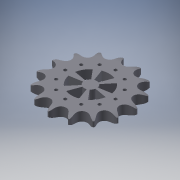
# Autodesk Inventor part: outer_drive_sprocket
Saved by Autodesk Inventor 2016 (Build 200138000, 138)
## iProperties
Created: 2016-11-04
Part Number: outer_drive_sprocket
Material: Steel
Document SubType Name: Modeling
Designer: hesaon
Density: 1 g/cm^3
Appearance: Steel
CustomPartVersion: 1
Author: hesaon
Autodesk Inventor part; units mm, degrees
ref_plane "YZ Plane" through (0, 0, 0) normal (1, 0, 0) x (0, 1, 0)
ref_plane "XZ Plane" through (0, 0, 0) normal (0, 1, 0) x (-1, 0, 0)
ref_plane "XY Plane" through (0, 0, 0) normal (0, 0, 1) x (1, 0, 0)
sketch "Theoretical Tooth Profile" plane through (0, 0, 0) normal (0, 0, 1) x (1, 0, 0)
  circle A0 centre (0, 0) radius 30.5418 construction
  line L0 (0, 0) -> (0, 30.5418) construction
  line L1 (0, 0) -> (12.4225, 27.9013) construction
  circle A1 centre (0, 0) radius 33.6844
  arc A2 (-3.3398, 27.8373) -> (3.3398, 27.8373) centre (0, 30.5418) ccw
  line L2 (0, 30.5418) -> (12.4225, 27.9013) construction
  line L3 (0, 30.5418) -> (5.2908, 34.8262) construction
  line L4 (5.2908, 34.8262) -> (-4.796, 30.1797) construction
  arc A3 (6.5675, 33.038) -> (5.1927, 31.041) centre (11.6537, 28.0648) ccw
  arc A4 (-5.1927, 31.041) -> (-6.5675, 33.038) centre (-11.6537, 28.0648) ccw
  line L5 (-11.6537, 28.0648) -> (-5.1927, 31.041) construction
  arc A5 (-4.796, 30.1797) -> (-3.3398, 27.8373) centre (5.2908, 34.8262) ccw
  line L6 (-4.796, 30.1797) -> (-5.1927, 31.041)
  arc A6 (3.3398, 27.8373) -> (4.796, 30.1797) centre (-5.2908, 34.8262) ccw
  line L7 (5.1927, 31.041) -> (4.796, 30.1797)
  line L8 (0, 0) -> (7.0034, 32.9483) construction
  point P0 (6.2112, 29.2216)
  dimension "d0" = 61.0836
  dimension "d2" = 24
  dimension "d3" = 4.2976
  dimension "d10" = 129
  dimension "d11" = 14.267
  dimension "d12" = 6.808
  dimension "d13" = 11.1055
  dimension "d14" = 11.914
  dimension "d23" = 3.81
  constraints: 18 end point, 15 point on circle, 7 centre point, 3 coincident, 3 point on line, 3 symmetric about line, 3 tangent, 1 equal radius, 1 midpoint, 1 parallel, 1 vertical, 1 other
  measures "d0" diameter of A0
  measures "d2" angle of L1 L0
  measures "d3" radius of A2
  measures "d10" angle of L3 L0
  measures "d11" angle of L4 L3
  measures "d12" distance of L2.start L3.end
  measures "d13" distance of L3.end L4.end
  measures "d14" distance of A3.centre L0.end
  measures "d23" distance from line of L8.end L2
sketch "Tooth Profile" plane through (0, 0, 0) normal (0, 0, 1) x (1, 0, 0)
  arc A0 (-3.9559, 28.8626) -> (3.9559, 28.8626) centre (0, 30.5418) ccw
  arc A1 (6.485, 33.0543) -> (3.9559, 28.8626) centre (19.9362, 22.0794) ccw
  arc A2 (-3.9559, 28.8626) -> (-6.485, 33.0543) centre (-19.9362, 22.0794) ccw
  line L0 (0, 0) -> (0, 30.5418) construction
  line L1 (0, 30.5418) -> (3.9559, 28.8626) construction
  line L2 (0, 30.5418) -> (-3.9559, 28.8626) construction
  circle A3 centre (0, 0) radius 33.6844 projected
  dimension "d44" = 134
  dimension "d45" = 17.3604
  dimension "d46" = 4.2976
  constraints: 9 point on circle, 6 end point, 3 centre point, 2 tangent, 1 coincident, 1 equal radius, 1 vertical, 1 other
  measures "d44" angle of L2 L1
  measures "d45" radius of A1
  measures "d46" radius of A0
sketch "Section Profile" plane through (0, 0, 0) normal (1, 0, 0) x (0, 1, 0)
  line L0 (33.6844, 0) -> (-33.6844, 0) projected
  line L1 (19.4252, 3.6038) -> (-19.4252, 3.6038)
  line L2 (-19.4252, 3.6038) -> (-19.4252, -3.6037)
  line L3 (-19.4252, -3.6037) -> (19.4252, -3.6037)
  line L4 (19.4252, -3.6037) -> (19.4252, 3.6038)
  line L5 (19.4252, 3.6037) -> (33.6844, 3.6037) construction
  line L6 (33.6844, 3.6037) -> (33.6844, -3.6037) construction
  line L7 (33.6844, -3.6037) -> (19.4252, -3.6037) construction
  line L8 (19.4252, -3.6037) -> (19.4252, 3.6037)
  arc A0 (33.6844, 2.0162) -> (27.536, 3.6037) centre (27.536, -9.0963) ccw
  arc A1 (27.536, -3.6037) -> (33.6844, -2.0162) centre (27.536, 9.0963) ccw
  line L9 (27.536, 3.6037) -> (0, 3.6037)
  line L10 (0, 3.6037) -> (0, -3.6037)
  line L11 (0, -3.6037) -> (27.536, -3.6037)
  line L12 (0, 3.6037) -> (0, -3.6037)
  line L13 (33.6844, 2.0162) -> (33.6844, -2.0162)
  point P0 (0, 0)
  point P1 (0, 0)
  dimension "d30" = 7.2075
  dimension "d31" = 38.8504
  dimension "d32" = 7.2075
  dimension "d33" = 1.5875
  dimension "d34" = 12.7
  dimension "d43" = 3.6037
  constraints: 26 end point, 7 midpoint, 5 perpendicular, 4 parallel, 4 point on circle, 3 point on line, 3 symmetric about line, 2 centre point, 2 horizontal, 2 tangent, 1 collinear, 1 other
  measures "d30" distance between parallel lines of L7 L5
  measures "d31" distance between parallel lines of L2 L4
  measures "d32" distance between parallel lines of L3 L1
  measures "d33" distance from line of L13.start L5
  measures "d34" radius of A0
  measures "d43" distance between parallel lines of L3 L0
revolve "Shroud" add sketch "Section Profile" angle 360 about axis through (0, 0, 3.6037) along (0, 0, -1) contours L10 L3 L2 L0 | L0 L2 L1 L10
revolve "Strand" add sketch "Section Profile" angle 360 about axis through (0, 0, 3.6037) along (0, 0, -1) contours L13 A1 L11 L4 L0 | L0 L4 L9 A0 L13 | L4 L3 L10 L0 | L0 L10 L1 L4
pattern_of_one "Strand Pattern"
extrude "Theoretical Tooth" cut sketch "Theoretical Tooth Profile" along normal through all both and the other way through all contours A3 L7 A6 A2 A5 L6 A4 A1 picked at (0, 31.1563)
extrude "Tooth" [suppressed]
pattern_circular "Tooth Pattern" count 15 over 360 about axis through (0, 0, -10) along (0, 0, 1) of "Theoretical Tooth"
ref_plane "Timing Plane" through (0, 30.5418, 0) normal (1, 0, 0) x (0, 1, 0)
sketch "Sketch4" plane through (0, 30.5418, 3.6038) normal (0, 0, 1) x (1, 0, 0)
  arc A0 (-26.9414, -24.8503) -> (-27.536, -30.5075) centre (0, -30.5418) ccw projected
  arc A1 (1.7101, -25.8433) -> (-1.7101, -25.8433) centre (0, -30.5418) ccw
  arc A2 (5.1303, -16.4464) -> (-5.1303, -16.4464) centre (0, -30.5418) ccw
  line L0 (-1.7101, -25.8433) -> (-5.1303, -16.4464)
  line L1 (1.7101, -25.8433) -> (5.1303, -16.4464)
  arc A3 (1.7101, -25.8433) -> (-1.7101, -25.8433) centre (0, -30.5418) ccw
  arc A4 (5.1303, -16.4464) -> (-5.1303, -16.4464) centre (0, -30.5418) ccw
  line L2 (-4.924, -29.6736) -> (-14.7721, -27.9371)
  arc A5 (-9.6418, -19.0511) -> (-14.7721, -27.9371) centre (0, -30.5418) ccw
  line L3 (-3.2139, -26.7116) -> (-9.6418, -19.0511)
  arc A6 (-3.2139, -26.7116) -> (-4.924, -29.6736) centre (0, -30.5418) ccw
  line L4 (-3.2139, -34.372) -> (-9.6418, -42.0325)
  arc A7 (-14.7721, -33.1465) -> (-9.6418, -42.0325) centre (0, -30.5418) ccw
  line L5 (-4.924, -31.4101) -> (-14.7721, -33.1465)
  arc A8 (-4.924, -31.4101) -> (-3.2139, -34.372) centre (0, -30.5418) ccw
  line L6 (1.7101, -35.2403) -> (5.1303, -44.6372)
  arc A9 (-5.1303, -44.6372) -> (5.1303, -44.6372) centre (0, -30.5418) ccw
  line L7 (-1.7101, -35.2403) -> (-5.1303, -44.6372)
  arc A10 (-1.7101, -35.2403) -> (1.7101, -35.2403) centre (0, -30.5418) ccw
  line L8 (4.924, -31.4101) -> (14.7721, -33.1465)
  arc A11 (9.6418, -42.0325) -> (14.7721, -33.1465) centre (0, -30.5418) ccw
  line L9 (3.2139, -34.372) -> (9.6418, -42.0325)
  arc A12 (3.2139, -34.372) -> (4.924, -31.4101) centre (0, -30.5418) ccw
  line L10 (3.2139, -26.7116) -> (9.6418, -19.0511)
  arc A13 (14.7721, -27.9371) -> (9.6418, -19.0511) centre (0, -30.5418) ccw
  line L11 (4.924, -29.6736) -> (14.7721, -27.9371)
  arc A14 (4.924, -29.6736) -> (3.2139, -26.7116) centre (0, -30.5418) ccw
  point P0 (0, -15.5418)
  point P1 (-12.9904, -23.0418)
  point P2 (-12.9904, -38.0418)
  point P3 (0, -45.5418)
  point P4 (12.9904, -38.0418)
  point P5 (12.9904, -23.0418)
  dimension "d88" = 10
  dimension "d89" = 30
  dimension "d95" = 360
  constraints: 29 point on circle, 24 end point, 14 centre point, 9 coincident, 67 other
  measures "d88" diameter of A1
  measures "d89" diameter of A2
extrude "Extrusion4" cut sketch "Sketch4" against normal through all
sketch "Sketch5" plane through (0, 30.5418, 3.6038) normal (0, 0, 1) x (1, 0, 0)
  circle A0 centre (-20, -30.5418) radius 1.25
  circle A1 centre (-17.3205, -40.5418) radius 1.25
  circle A2 centre (-10, -47.8623) radius 1.25
  circle A3 centre (0, -50.5418) radius 1.25
  circle A4 centre (10, -47.8623) radius 1.25
  circle A5 centre (17.3205, -40.5418) radius 1.25
  circle A6 centre (20, -30.5418) radius 1.25
  circle A7 centre (17.3205, -20.5418) radius 1.25
  circle A8 centre (10, -13.2213) radius 1.25
  circle A9 centre (0, -10.5418) radius 1.25
  circle A10 centre (-10, -13.2213) radius 1.25
  circle A11 centre (-17.3205, -20.5418) radius 1.25
  point P0 (0, -30.5418)
  dimension "d100" = 2.5
  dimension "d103" = 360
  dimension "d105" = 20
  constraints: 12 centre point, 25 other
  measures "d100" diameter of A0
  measures "d105" distance of point (0, -30.542) A0.centre
extrude "Extrusion5" cut sketch "Sketch5" against normal through all
equation "\"d3\" = 0.5 * da_Dr + da_SC"
equation "\"d12\" = 0.8 * da_Dr"
equation "\"d13\" = 1.3 * da_Dr + da_SC"
equation "\"d14\" = 1.4 * da_Dr"
equation "\"d23\" = da_Ha"
equation "\"d44\" = da_Alfa"
equation "\"d45\" = da_Re"
equation "\"d46\" = da_Ri"
equation "\"d30\" = da_Bf"
equation "\"d31\" = da_Ds"
equation "\"d32\" = da_Bs"
equation "\"d33\" = da_Ba"
equation "\"d34\" = da_Rx"
equation "\"d40\" = da_pt"
equation "\"form_type\" = 0"
equation "\"da_p\" = 12.7"
equation "\"da_Dr\" = 8.51"
equation "\"da_SC\" = 0.04255"
equation "\"da_Ha\" = 3.81"
equation "\"da_pt\" = 13.92"
equation "\"da_Bf\" = 7.2075"
equation "\"da_Ba\" = 1.5875"
equation "\"da_Rx\" = 12.7"
equation "\"da_Ra\" = 0.508"
equation "\"da_Bs\" = 7.2075"
equation "\"da_Ds\" = 38.8504"
equation "\"da_Re\" = 17.3604"
equation "\"da_Ri\" = 4.29755"
equation "\"da_Alfa\" = 134deg"
body "Solid1"
